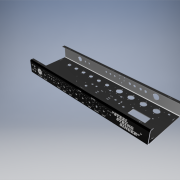
# Autodesk Inventor part: Main Enclosurewith silkscreen
Saved by Autodesk Inventor 2018.1 (Build 221171000, 171)
## iProperties
Created: 2017-10-21
Part Number: Main Enclosurewith silkscreen
Material: Aluminum 6061
Document SubType Name: Sheet Metal
Designer: RCCol
Density: 2.7 g/cm^3
Sheet Metal Rule: .125 thick aluminum
Appearance: Aluminum - Flat
Sheet Metal Width: 14.631 in
Sheet Metal Length: 26.500 in
Sheet Metal Area: 387.721 in^2
Flat Pattern Width: 37.1627 cm
Flat Pattern Length: 67.31 cm
Flat Pattern Area: 2501.42 cm^2
Author: RCCol
Autodesk Inventor part; units mm, degrees
ref_plane "YZ Plane" through (0, 0, 0) normal (1, 0, 0) x (0, 1, 0)
ref_plane "XZ Plane" through (0, 0, 0) normal (0, 1, 0) x (-1, 0, 0)
ref_plane "XY Plane" through (0, 0, 0) normal (0, 0, 1) x (1, 0, 0)
sketch "Sketch2" plane through (0, 0, 0) normal (0, 1, 0) x (-1, 0, 0)
  circle A0 centre (244.7036, -254.3608) radius 1.651
  circle A1 centre (234.6008, -260.133) radius 1.651
  circle A2 centre (193.9036, -270.2358) radius 9.525
  circle A3 centre (140.559, -225.1508) radius 1.65
  line L0 (-268.3747, -289.9675) -> (-268.3747, -293.6791)
  arc A4 (-268.3747, -289.9675) -> (-268.97, -289.3722) centre (-268.97, -289.9675) ccw
  line L1 (-271.0814, -289.3722) -> (-268.97, -289.3722)
  arc A5 (-271.0814, -289.3722) -> (-271.6767, -289.9675) centre (-271.0814, -289.9675) ccw
  line L2 (-271.6767, -293.6791) -> (-271.6767, -289.9675)
  arc A6 (-271.6767, -293.6791) -> (-271.0814, -294.2744) centre (-271.0814, -293.6791) ccw
  line L3 (-268.97, -294.2744) -> (-271.0814, -294.2744)
  arc A7 (-268.97, -294.2744) -> (-268.3747, -293.6791) centre (-268.97, -293.6791) ccw
  circle A8 centre (-298.0757, -244.2954) radius 1.651
  circle A9 centre (143.1036, -270.2358) radius 9.525
  line L4 (-268.3747, -249.9675) -> (-268.3747, -253.6791)
  arc A10 (-268.3747, -249.9675) -> (-268.97, -249.3722) centre (-268.97, -249.9675) ccw
  line L5 (-271.0814, -249.3722) -> (-268.97, -249.3722)
  arc A11 (-271.0814, -249.3722) -> (-271.6767, -249.9675) centre (-271.0814, -249.9675) ccw
  line L6 (-271.6767, -253.6791) -> (-271.6767, -249.9675)
  arc A12 (-271.6767, -253.6791) -> (-271.0814, -254.2744) centre (-271.0814, -253.6791) ccw
  line L7 (-268.97, -254.2744) -> (-271.0814, -254.2744)
  arc A13 (-268.97, -254.2744) -> (-268.3747, -253.6791) centre (-268.97, -253.6791) ccw
  circle A14 centre (143.1036, -254.3608) radius 1.651
  circle A15 centre (-285.3757, -224.1983) radius 3.175
  circle A16 centre (133.0008, -260.133) radius 1.651
  circle A17 centre (92.3036, -286.1108) radius 1.651
  circle A18 centre (202.3125, -144.8233) radius 1.651
  circle A19 centre (71.2868, -214.9908) radius 2.3813
  circle A20 centre (-285.3757, -147.9983) radius 3.175
  circle A21 centre (190.3125, -135.2983) radius 1.651
  circle A22 centre (92.3036, -254.3608) radius 1.651
  circle A23 centre (-174.7757, -281.3483) radius 1.651
  circle A24 centre (176.9125, -135.2983) radius 1.651
  circle A25 centre (42.134, -229.1208) radius 4.826
  arc A26 (-141.3747, -289.9675) -> (-141.97, -289.3722) centre (-141.97, -289.9675) ccw
  line L8 (-144.0814, -289.3722) -> (-141.97, -289.3722)
  arc A27 (-144.0814, -289.3722) -> (-144.6767, -289.9675) centre (-144.0814, -289.9675) ccw
  line L9 (-144.6767, -293.6791) -> (-144.6767, -289.9675)
  arc A28 (-144.6767, -293.6791) -> (-144.0814, -294.2744) centre (-144.0814, -293.6791) ccw
  line L10 (-141.97, -294.2744) -> (-144.0814, -294.2744)
  arc A29 (-141.97, -294.2744) -> (-141.3747, -293.6791) centre (-141.97, -293.6791) ccw
  line L11 (-141.3747, -289.9675) -> (-141.3747, -293.6791)
  circle A30 centre (157.8625, -135.2983) radius 1.651
  circle A31 centre (41.5036, -270.2358) radius 9.525
  circle A32 centre (16.734, -229.1208) radius 4.826
  circle A33 centre (-111.2757, -280.4425) radius 1.651
  circle A34 centre (-47.7757, -280.4425) radius 1.651
  circle A35 centre (-190.1257, -224.1983) radius 3.175
  arc A36 (-141.3747, -249.9675) -> (-141.97, -249.3722) centre (-141.97, -249.9675) ccw
  line L12 (-144.0814, -249.3722) -> (-141.97, -249.3722)
  arc A37 (-144.0814, -249.3722) -> (-144.6767, -249.9675) centre (-144.0814, -249.9675) ccw
  line L13 (-144.6767, -253.6791) -> (-144.6767, -249.9675)
  arc A38 (-144.6767, -253.6791) -> (-144.0814, -254.2744) centre (-144.0814, -253.6791) ccw
  line L14 (-141.97, -254.2744) -> (-144.0814, -254.2744)
  arc A39 (-141.97, -254.2744) -> (-141.3747, -253.6791) centre (-141.97, -253.6791) ccw
  line L15 (-141.3747, -249.9675) -> (-141.3747, -253.6791)
  circle A40 centre (-19.3992, -260.133) radius 1.651
  circle A41 centre (-79.5257, -271.8233) radius 15.1
  line L16 (-28.621, -217.7185) -> (-21.621, -217.7185)
  arc A42 (-28.621, -217.7185) -> (-28.621, -222.7185) centre (-28.621, -220.2185) ccw
  line L17 (-21.621, -222.7185) -> (-28.621, -222.7185)
  arc A43 (-21.621, -222.7185) -> (-21.621, -217.7185) centre (-21.621, -220.2185) ccw
  arc A44 (-77.8747, -249.9675) -> (-78.47, -249.3722) centre (-78.47, -249.9675) ccw
  line L18 (-80.5814, -249.3722) -> (-78.47, -249.3722)
  arc A45 (-80.5814, -249.3722) -> (-81.1767, -249.9675) centre (-80.5814, -249.9675) ccw
  line L19 (-81.1767, -253.6791) -> (-81.1767, -249.9675)
  arc A46 (-81.1767, -253.6791) -> (-80.5814, -254.2744) centre (-80.5814, -253.6791) ccw
  line L20 (-78.47, -254.2744) -> (-80.5814, -254.2744)
  arc A47 (-78.47, -254.2744) -> (-77.8747, -253.6791) centre (-78.47, -253.6791) ccw
  line L21 (-77.8747, -249.9675) -> (-77.8747, -253.6791)
  circle A48 centre (-99.2757, -246.7925) radius 1.65
  circle A49 centre (-35.7757, -248.38) radius 1.65
  circle A50 centre (-60.681, -232.1358) radius 1.65
  circle A51 centre (-47.7757, -248.38) radius 4.826
  circle A52 centre (-172.441, -232.1358) radius 1.65
  circle A53 centre (-10.2592, -172.0483) radius 6.35
  circle A54 centre (-83.8585, -220.2185) radius 2.65
  line L22 (-83.768, -202.6483) -> (-76.768, -202.6483)
  arc A55 (-83.768, -202.6483) -> (-83.768, -207.6483) centre (-83.768, -205.1483) ccw
  line L23 (-76.768, -207.6483) -> (-83.768, -207.6483)
  arc A56 (-76.768, -207.6483) -> (-76.768, -202.6483) centre (-76.768, -205.1483) ccw
  line L24 (-18.6805, -126.4483) -> (-11.6805, -126.4483)
  arc A57 (-18.6805, -126.4483) -> (-18.6805, -131.4483) centre (-18.6805, -128.9483) ccw
  line L25 (-11.6805, -131.4483) -> (-18.6805, -131.4483)
  arc A58 (-11.6805, -131.4483) -> (-11.6805, -126.4483) centre (-11.6805, -128.9483) ccw
  line L26 (-28.621, -135.1685) -> (-21.621, -135.1685)
  arc A59 (-28.621, -135.1685) -> (-28.621, -140.1685) centre (-28.621, -137.6685) ccw
  line L27 (-21.621, -140.1685) -> (-28.621, -140.1685)
  arc A60 (-21.621, -140.1685) -> (-21.621, -135.1685) centre (-21.621, -137.6685) ccw
  circle A61 centre (-160.0585, -201.043) radius 4.8
  circle A62 centre (-60.681, -143.2358) radius 1.65
  circle A63 centre (-134.6585, -168.6358) radius 2.65
  circle A64 centre (-172.441, -143.2358) radius 1.65
  line L28 (-83.768, -126.4483) -> (-76.768, -126.4483)
  arc A65 (-83.768, -126.4483) -> (-83.768, -131.4483) centre (-83.768, -128.9483) ccw
  line L29 (-76.768, -131.4483) -> (-83.768, -131.4483)
  arc A66 (-76.768, -131.4483) -> (-76.768, -126.4483) centre (-76.768, -128.9483) ccw
  circle A67 centre (-134.6585, -128.9483) radius 2.65
  line L30 (-132.1585, -137.9577) -> (-132.1585, -142.9577)
  arc A68 (-132.1585, -137.9577) -> (-137.1585, -137.9577) centre (-134.6585, -137.9577) ccw
  line L31 (-137.1585, -142.9577) -> (-137.1585, -137.9577)
  arc A69 (-137.1585, -142.9577) -> (-132.1585, -142.9577) centre (-134.6585, -142.9577) ccw
  circle A70 centre (-83.8585, -137.6685) radius 2.65
  circle A71 centre (-75.921, -137.6685) radius 2.65
  circle A72 centre (-85.1892, -172.0483) radius 6.35
  line L32 (-132.1585, -202.9264) -> (-132.1585, -207.9264)
  arc A73 (-132.1585, -202.9264) -> (-137.1585, -202.9264) centre (-134.6585, -202.9264) ccw
  line L33 (-137.1585, -207.9264) -> (-137.1585, -202.9264)
  arc A74 (-137.1585, -207.9264) -> (-132.1585, -207.9264) centre (-134.6585, -207.9264) ccw
  line L34 (-83.768, -191.9483) -> (-76.768, -191.9483)
  arc A75 (-83.768, -191.9483) -> (-83.768, -196.9483) centre (-83.768, -194.4483) ccw
  line L35 (-76.768, -196.9483) -> (-83.768, -196.9483)
  arc A76 (-76.768, -196.9483) -> (-76.768, -191.9483) centre (-76.768, -194.4483) ccw
  circle A77 centre (-40.416, -168.0008) radius 1.65
  circle A78 centre (-107.616, -213.8685) radius 4.8
  line L36 (-132.1585, -216.9358) -> (-132.1585, -221.9358)
  arc A79 (-132.1585, -216.9358) -> (-137.1585, -216.9358) centre (-134.6585, -216.9358) ccw
  line L37 (-137.1585, -221.9358) -> (-137.1585, -216.9358)
  arc A80 (-137.1585, -221.9358) -> (-132.1585, -221.9358) centre (-134.6585, -221.9358) ccw
  circle A81 centre (-75.921, -220.2185) radius 2.65
  circle A82 centre (-190.1257, -147.9983) radius 3.175
  line L38 (-18.6805, -191.9483) -> (-11.6805, -191.9483)
  arc A83 (-18.6805, -191.9483) -> (-18.6805, -196.9483) centre (-18.6805, -194.4483) ccw
  line L39 (-11.6805, -196.9483) -> (-18.6805, -196.9483)
  arc A84 (-11.6805, -196.9483) -> (-11.6805, -191.9483) centre (-11.6805, -194.4483) ccw
  line L40 (-196.4757, -155.6433) -> (-196.4757, -216.5533)
  arc A85 (-196.4757, -155.6433) -> (-199.6757, -152.4433) centre (-199.6757, -155.6433) ccw
  line L41 (-275.8257, -152.4433) -> (-199.6757, -152.4433)
  arc A86 (-275.8257, -152.4433) -> (-279.0257, -155.6433) centre (-275.8257, -155.6433) ccw
  line L42 (-279.0257, -216.5533) -> (-279.0257, -155.6433)
  arc A87 (-279.0257, -216.5533) -> (-275.8257, -219.7533) centre (-275.8257, -216.5533) ccw
  line L43 (-199.6757, -219.7533) -> (-275.8257, -219.7533)
  arc A88 (-199.6757, -219.7533) -> (-196.4757, -216.5533) centre (-199.6757, -216.5533) ccw
  circle A89 centre (-59.7757, -248.38) radius 1.65
  line L44 (-18.6805, -202.6483) -> (-11.6805, -202.6483)
  arc A90 (-18.6805, -202.6483) -> (-18.6805, -207.6483) centre (-18.6805, -205.1483) ccw
  line L45 (-11.6805, -207.6483) -> (-18.6805, -207.6483)
  arc A91 (-11.6805, -207.6483) -> (-11.6805, -202.6483) centre (-11.6805, -205.1483) ccw
  circle A92 centre (-111.2757, -246.7925) radius 4.826
  circle A93 centre (-40.416, -225.1508) radius 1.65
  circle A94 centre (-123.2757, -246.7925) radius 1.65
  circle A95 centre (-9.2964, -254.3608) radius 1.651
  circle A96 centre (-9.2964, -270.2358) radius 9.525
  circle A97 centre (-143.0257, -271.8233) radius 15.1
  circle A98 centre (144.4625, -135.2983) radius 1.651
  circle A99 centre (31.4008, -260.133) radius 1.651
  circle A100 centre (-179.9657, -245.0256) radius 1.651
  circle A101 centre (0.8064, -280.3386) radius 1.651
  arc A102 (-77.8747, -289.9675) -> (-78.47, -289.3722) centre (-78.47, -289.9675) ccw
  line L46 (-80.5814, -289.3722) -> (-78.47, -289.3722)
  arc A103 (-80.5814, -289.3722) -> (-81.1767, -289.9675) centre (-80.5814, -289.9675) ccw
  line L47 (-81.1767, -293.6791) -> (-81.1767, -289.9675)
  arc A104 (-81.1767, -293.6791) -> (-80.5814, -294.2744) centre (-80.5814, -293.6791) ccw
  line L48 (-78.47, -294.2744) -> (-80.5814, -294.2744)
  arc A105 (-78.47, -294.2744) -> (-77.8747, -293.6791) centre (-78.47, -293.6791) ccw
  line L49 (-77.8747, -289.9675) -> (-77.8747, -293.6791)
  circle A106 centre (53.7855, -199.9147) radius 6.35
  line L50 (-204.8747, -249.9675) -> (-204.8747, -253.6791)
  arc A107 (-204.8747, -249.9675) -> (-205.47, -249.3722) centre (-205.47, -249.9675) ccw
  line L51 (-207.5814, -249.3722) -> (-205.47, -249.3722)
  arc A108 (-207.5814, -249.3722) -> (-208.1767, -249.9675) centre (-207.5814, -249.9675) ccw
  line L52 (-208.1767, -253.6791) -> (-208.1767, -249.9675)
  arc A109 (-208.1767, -253.6791) -> (-207.5814, -254.2744) centre (-207.5814, -253.6791) ccw
  line L53 (-205.47, -254.2744) -> (-207.5814, -254.2744)
  arc A110 (-205.47, -254.2744) -> (-204.8747, -253.6791) centre (-205.47, -253.6791) ccw
  circle A111 centre (-206.5257, -271.8233) radius 15.1
  circle A112 centre (51.6064, -280.3386) radius 1.651
  circle A113 centre (82.2008, -260.133) radius 1.651
  circle A114 centre (92.3036, -270.2358) radius 9.525
  circle A115 centre (-285.3757, -129.8538) radius 1.5
  circle A116 centre (-238.2757, -244.2954) radius 1.651
  line L54 (-204.8747, -289.9675) -> (-204.8747, -293.6791)
  arc A117 (-204.8747, -289.9675) -> (-205.47, -289.3722) centre (-205.47, -289.9675) ccw
  line L55 (-207.5814, -289.3722) -> (-205.47, -289.3722)
  arc A118 (-207.5814, -289.3722) -> (-208.1767, -289.9675) centre (-207.5814, -289.9675) ccw
  line L56 (-208.1767, -293.6791) -> (-208.1767, -289.9675)
  arc A119 (-208.1767, -293.6791) -> (-207.5814, -294.2744) centre (-207.5814, -293.6791) ccw
  line L57 (-205.47, -294.2744) -> (-207.5814, -294.2744)
  arc A120 (-205.47, -294.2744) -> (-204.8747, -293.6791) centre (-205.47, -293.6791) ccw
  circle A121 centre (98.653, -179.9637) radius 2.3813
  circle A122 centre (102.4064, -280.3386) radius 1.651
  circle A123 centre (-238.2757, -280.4425) radius 1.651
  circle A124 centre (110.892, -194.8109) radius 2.3813
  circle A125 centre (-270.0257, -271.8233) radius 15.1
  circle A126 centre (221.3625, -144.8233) radius 1.651
  circle A127 centre (140.559, -168.0008) radius 1.65
  circle A128 centre (153.2064, -280.3386) radius 1.651
  circle A129 centre (183.8008, -260.133) radius 1.651
  circle A130 centre (-294.9007, -286.7925) radius 1.651
  circle A131 centre (204.0064, -280.3386) radius 1.651
  circle A132 centre (244.7036, -270.2358) radius 9.525
  circle A133 centre (254.8064, -280.3386) radius 1.651
  line L58 (322.2625, -312.7375) -> (-350.8375, -312.7375)
  line L59 (-350.8375, -312.7375) -> (-350.8375, -96.8375)
  line L60 (-350.8375, -96.8375) -> (322.2625, -96.8375)
  line L61 (322.2625, -96.8375) -> (322.2625, -312.7375)
  circle A134 centre (317.5, -133.35) radius 2.667
  circle A135 centre (317.5, -140.6906) radius 1.5875
  circle A136 centre (317.5, -126.0094) radius 1.5875
  circle A137 centre (317.5, -273.05) radius 2.667
  circle A138 centre (317.5, -280.3906) radius 1.5875
  circle A139 centre (317.5, -265.7094) radius 1.5875
  point P0 (0, 0)
  dimension "d2" = 673.1
  dimension "d3" = 215.9
  measures "d2" distance of L59.end L60.end
  measures "d3" distance of L58.end L59.end
extrude "Plate1" add sketch "Sketch2" along normal blind 3.175 contours L58 L59 L60 L61 | A134 | A135 | A136 | A137 | A138 | A139
sketch "Sketch3" plane through (350.8375, 0, -100.0125) normal (0, 0, 1) x (1, 0, 0)
  line L0 (-673.1, 0) -> (0, 0)
  line L1 (0, 0) -> (0, 69.85)
  line L2 (0, 69.85) -> (-673.1, 69.85)
  line L3 (-673.1, 69.85) -> (-673.1, 0)
  constraints: 6 end point, 1 horizontal, 1 perpendicular, 1 vertical
edge flange "Flange1" height 69.85 angle 90 thickness 3.175 bend radius 3.175 thickness toward (0, 0, 1) relief tear relief width 3.175 relief depth 1.5875 edges at (14.2875, 3.175, -96.8375) wall of the first edge with corners at (-322.2625, 0, -100.0125) (350.8375, 0, -100.0125) (350.8375, 69.85, -100.0125) (-322.2625, 69.85, -100.0125)
bend "Bend1"
corner "Corner1"
sketch "Sketch4" plane through (-322.2625, 0, -309.5625) normal (0, 0, -1) x (-1, 0, 0)
  line L0 (-673.1, 0) -> (0, 0)
  line L1 (0, 0) -> (0, 69.85)
  line L2 (0, 69.85) -> (-673.1, 69.85)
  line L3 (-673.1, 69.85) -> (-673.1, 0)
  constraints: 6 end point, 1 horizontal, 1 perpendicular, 1 vertical
edge flange "Flange2" height 69.85 angle 90 thickness 3.175 bend radius 3.175 thickness toward (0, 0, -1) relief tear relief width 3.175 relief depth 1.5875 edges at (14.2875, 3.175, -312.7375) wall of the first edge with corners at (350.8375, 0, -309.5625) (-322.2625, 0, -309.5625) (-322.2625, 69.85, -309.5625) (350.8375, 69.85, -309.5625)
bend "Bend2"
corner "Corner2"
sketch "A$C2850429B" plane through (0, 0, 0) normal (0, 0, 1) x (1, 0, 0)
  circle A0 centre (0, 0) radius 1.778
sketch "A$C2850429B_1" plane through (0, 0, 0) normal (0, 0, 1) x (1, 0, 0)
  circle A0 centre (0, 0) radius 1.778
sketch "A$C2850429B_2" plane through (0, 0, 0) normal (0, 0, 1) x (1, 0, 0)
  circle A0 centre (0, 0) radius 1.778
sketch "Sketch9" plane through (-322.2625, 69.85, -96.8375) normal (0, 0, 1) x (1, 0, 0)
  circle A0 centre (31.75, -22.225) radius 4.7625
  circle A1 centre (69.85, -34.925) radius 4.7625
  circle A2 centre (139.7, -34.925) radius 3.175
  circle A3 centre (171.704, -34.925) radius 3.175
  circle A4 centre (241.3, -34.925) radius 4.7625
  circle A5 centre (641.35, -34.925) radius 3.9624
  circle A6 centre (355.6, -34.925) radius 4.7625
  circle A7 centre (501.65, -34.925) radius 3.175
  circle A8 centre (469.9, -34.925) radius 4.7625
  circle A9 centre (431.8, -34.925) radius 4.7625
  circle A10 centre (393.7, -34.925) radius 4.7625
  circle A11 centre (317.5, -34.925) radius 4.7625
  circle A12 centre (279.4, -34.925) radius 4.7625
  circle A13 centre (203.2, -34.925) radius 4.7625
  circle A14 centre (155.702, -34.925) radius 3.175
  circle A15 centre (107.95, -34.925) radius 4.7625
  circle A16 centre (31.75, -47.625) radius 4.7625
  circle A17 centre (31.75, -47.625) radius 4.7625
  circle A18 centre (107.95, -34.925) radius 4.7625
  circle A19 centre (155.702, -34.925) radius 3.175
  circle A20 centre (203.2, -34.925) radius 4.7625
  circle A21 centre (279.4, -34.925) radius 4.7625
  circle A22 centre (317.5, -34.925) radius 4.7625
  circle A23 centre (393.7, -34.925) radius 4.7625
  circle A24 centre (431.8, -34.925) radius 4.7625
  circle A25 centre (469.9, -34.925) radius 4.7625
  circle A26 centre (501.65, -34.925) radius 3.175
  circle A27 centre (355.6, -34.925) radius 4.7625
  circle A28 centre (641.35, -34.925) radius 3.9624
  circle A29 centre (241.3, -34.925) radius 4.7625
  circle A30 centre (171.704, -34.925) radius 3.175
  circle A31 centre (139.7, -34.925) radius 3.175
  circle A32 centre (69.85, -34.925) radius 4.7625
  circle A33 centre (31.75, -22.225) radius 4.7625
  line L0 (0, -63.5) -> (0, 0) projected
  line L1 (0, -6.35) -> (673.1013, -6.35) construction
  line L2 (673.1013, -6.35) -> (673.1013, -63.5001) construction
  line L3 (673.1013, -63.5001) -> (0, -63.5001) construction
  line L4 (0, -63.5001) -> (0, -6.35) construction
  point P0 (322.2625, -69.85)
  constraints: 34 centre point, 17 concentric, 14 equal radius, 1 point on line, 2 other
extrude "Cut1" cut sketch "Sketch9" against normal blind 3.175
sketch "Sketch10" plane through (-322.2625, 69.85, -312.7375) normal (0, 1, 0) x (1, 0, 0)
  point P0 (322.2625, -312.7375)
sketch "Sketch13" plane through (-322.2625, 66.675, -312.7375) normal (0, 1, 0) x (-1, 0, 0)
  line L0 (-673.1, 0) -> (0, 0)
  line L1 (0, 0) -> (0, 19.05)
  line L2 (0, 19.05) -> (-673.1, 19.05)
  line L3 (-673.1, 19.05) -> (-673.1, 0)
  constraints: 6 end point, 1 horizontal, 1 perpendicular, 1 vertical
edge flange "Flange9" height 19.05 angle 90 thickness 3.175 bend radius 3.175 thickness toward (0, 1, 0) relief tear relief width 3.175 relief depth 1.5875 edges at (14.2875, 69.85, -309.5625) wall of the first edge with corners at (350.8375, 66.675, -312.7375) (-322.2625, 66.675, -312.7375) (-322.2625, 66.675, -293.6875) (350.8375, 66.675, -293.6875)
bend "Bend9"
corner "Corner9"
sketch "Sketch14" plane through (350.8375, 66.675, -96.8375) normal (0, 1, 0) x (-1, 0, 0)
  line L0 (673.1, 0) -> (0, 0)
  line L1 (0, 0) -> (0, -19.05)
  line L2 (0, -19.05) -> (673.1, -19.05)
  line L3 (673.1, -19.05) -> (673.1, 0)
  constraints: 6 end point, 1 horizontal, 1 perpendicular, 1 vertical
edge flange "Flange10" height 19.05 angle 90 thickness 3.175 bend radius 3.175 thickness toward (0, 1, 0) relief tear relief width 3.175 relief depth 1.5875 edges at (14.2875, 69.85, -100.0125) wall of the first edge with corners at (-322.2625, 66.675, -96.8375) (350.8375, 66.675, -96.8375) (350.8375, 66.675, -115.8875) (-322.2625, 66.675, -115.8875)
bend "Bend10"
corner "Corner10"
sketch "Sketch16" plane through (350.4375, 76.9937, -312.7375) normal (0, 0, -1) x (-1, 0, 0)
  line L0 (222.9999, -47.2355) -> (221.4962, -47.2355)
  arc A0 (222.9999, -48.2515) -> (221.4962, -48.2515) centre (222.248, -42.0741) ccw
  line L1 (221.4962, -47.2355) -> (221.4962, -48.2515)
  line L2 (222.9999, -48.2515) -> (222.9999, -47.2355)
  circle A1 centre (279.3859, -41.5187) radius 3.2385
  circle A2 centre (304.7859, -25.6437) radius 3.2385
  circle A3 centre (279.3859, -25.6437) radius 3.2385
  circle A4 centre (304.7859, -41.5187) radius 3.2385
  circle A5 centre (292.0309, -57.3937) radius 3.2385
  line L3 (196.213, -45.3834) -> (196.213, -38.7648)
  line L4 (184.783, -45.3834) -> (184.783, -38.7648)
  arc A6 (184.783, -45.3834) -> (196.213, -45.3834) centre (190.498, -42.0741) ccw
  arc A7 (196.213, -38.7648) -> (184.783, -38.7648) centre (190.498, -42.0741) ccw
  circle A8 centre (114.298, -42.0741) radius 14.7574
  circle A9 centre (135.253, -42.0741) radius 1.778
  circle A10 centre (93.343, -42.0741) radius 1.778
  line L5 (170.813, -45.3834) -> (170.813, -38.7648)
  line L6 (159.383, -45.3834) -> (159.383, -38.7648)
  arc A11 (159.383, -45.3834) -> (170.813, -45.3834) centre (165.098, -42.0741) ccw
  arc A12 (170.813, -38.7648) -> (159.383, -38.7648) centre (165.098, -42.0741) ccw
  line L7 (248.3999, -47.2355) -> (246.8962, -47.2355)
  arc A13 (248.3999, -48.2515) -> (246.8962, -48.2515) centre (247.648, -42.0741) ccw
  line L8 (246.8962, -47.2355) -> (246.8962, -48.2515)
  line L9 (248.3999, -48.2515) -> (248.3999, -47.2355)
  circle A14 centre (333.375, -41.5187) radius 4.7625
  circle A15 centre (358.775, -41.5187) radius 4.7625
  circle A16 centre (384.175, -41.5187) radius 4.7625
  circle A17 centre (495.2698, -42.1586) radius 4.7625
  circle A18 centre (520.6698, -42.1586) radius 4.7625
  circle A19 centre (558.7698, -42.1586) radius 12.1031
  circle A20 centre (545.9682, -34.7164) radius 1.778
  circle A21 centre (571.5714, -34.7164) radius 1.778
  circle A22 centre (558.7698, -56.9668) radius 1.778
  line L10 (-0.4, -13.4937) -> (672.6999, -13.4937) projected
  line L11 (-0.4, -13.4937) -> (672.7013, -13.4937) construction
  line L12 (672.7013, -13.4937) -> (672.7013, -70.6439) construction
  line L13 (672.7013, -70.6439) -> (-0.4, -70.6439) construction
  line L14 (-0.4, -70.6439) -> (-0.4, -13.4937) construction
  point P0 (322.2625, -69.85)
  constraints: 23 centre point, 20 end point, 14 equal radius, 12 point on circle, 2 concentric, 2 other
extrude "Cut2" cut sketch "Sketch16" against normal blind 3.175
sketch "Sketch17" plane through (-322.2625, 69.85, -293.6875) normal (0, 1, 0) x (1, 0, 0)
  circle A0 centre (50.8, -184.15) radius 2.667
  circle A1 centre (58.1406, -184.15) radius 1.5875
  circle A2 centre (43.4594, -184.15) radius 1.5875
  circle A3 centre (336.55, -184.15) radius 2.667
  circle A4 centre (343.8906, -184.15) radius 1.5875
  circle A5 centre (329.2094, -184.15) radius 1.5875
  circle A6 centre (622.3, -184.15) radius 2.667
  circle A7 centre (629.6406, -184.15) radius 1.5875
  circle A8 centre (614.9594, -184.15) radius 1.5875
  point P0 (322.2625, -293.6875)
  constraints: 9 centre point, 7 equal radius
extrude "Cut3" cut sketch "Sketch17" against normal blind 3.175
sketch "Sketch18" plane through (-322.2625, 69.85, -293.6875) normal (0, 1, 0) x (1, 0, 0)
  circle A0 centre (50.8, 6.35) radius 2.667
  circle A1 centre (58.1406, 6.35) radius 1.5875
  circle A2 centre (43.4594, 6.35) radius 1.5875
  circle A3 centre (336.55, 6.35) radius 2.667
  circle A4 centre (343.8906, 6.35) radius 1.5875
  circle A5 centre (329.2094, 6.35) radius 1.5875
  circle A6 centre (622.3, 6.35) radius 2.667
  circle A7 centre (629.6406, 6.35) radius 1.5875
  circle A8 centre (614.9594, 6.35) radius 1.5875
  point P0 (322.2625, -293.6875)
  constraints: 9 centre point, 7 equal radius
extrude "Cut4" cut sketch "Sketch18" against normal blind 3.175
sketch "Sketch21" plane through (0, 3.175, 0) normal (0, 1, 0) x (1, 0, 0)
  point P0 (0, 0)
sketch "Sketch22" plane through (0, 3.175, 0) normal (0, 1, 0) x (1, 0, 0)
  circle A0 centre (342.9, 274.6375) radius 2.667
  circle A1 centre (342.9, 267.2969) radius 1.5875
  circle A2 centre (342.9, 281.9781) radius 1.5875
  circle A3 centre (342.9, 134.9375) radius 2.667
  circle A4 centre (342.9, 127.5969) radius 1.5875
  circle A5 centre (342.9, 142.2781) radius 1.5875
  circle A6 centre (-314.325, 274.6375) radius 2.667
  circle A7 centre (-314.325, 267.2969) radius 1.5875
  circle A8 centre (-314.325, 281.9781) radius 1.5875
  circle A9 centre (-314.325, 134.9375) radius 2.667
  circle A10 centre (-314.325, 127.5969) radius 1.5875
  circle A11 centre (-314.325, 142.2781) radius 1.5875
  circle A12 centre (315.9125, 288.925) radius 4.7625
  point P0 (0, 0)
  dimension "BendReliefDepth" = 1.5875
  constraints: 13 centre point
extrude "Cut6" cut sketch "Sketch22" against normal blind 3.175
decal "Decal1"
decal "Decal2"
equation "\"d65\" = Thickness"
equation "\"BendReliefDepth\" = 0.5 * Thickness"
equation "\"d4\" = Thickness"
equation "\"d5\" = BendReliefWidth"
equation "\"d6\" = BendReliefDepth"
equation "\"d7\" = MinimumRemnant"
equation "\"d8\" = TransitionRadius"
equation "\"d11\" = BendRadius"
equation "\"d12\" = CornerReliefSize"
equation "\"d13\" = GapSize"
equation "\"d14\" = JacobiRadiusSize"
equation "\"d15\" = BendReliefWidth"
equation "\"d16\" = BendReliefDepth"
equation "\"d17\" = MinimumRemnant"
equation "\"d18\" = TransitionRadius"
equation "\"d21\" = BendRadius"
equation "\"d22\" = CornerReliefSize"
equation "\"d23\" = GapSize"
equation "\"d24\" = JacobiRadiusSize"
equation "\"d87\" = BendReliefWidth"
equation "\"d88\" = BendReliefDepth"
equation "\"d89\" = MinimumRemnant"
equation "\"d90\" = TransitionRadius"
equation "\"d93\" = BendRadius"
equation "\"d94\" = CornerReliefSize"
equation "\"d95\" = GapSize"
equation "\"d96\" = JacobiRadiusSize"
equation "\"d97\" = BendReliefWidth"
equation "\"d98\" = BendReliefDepth"
equation "\"d99\" = MinimumRemnant"
equation "\"d100\" = TransitionRadius"
equation "\"d103\" = BendRadius"
equation "\"d104\" = CornerReliefSize"
equation "\"d105\" = GapSize"
equation "\"d106\" = JacobiRadiusSize"
equation "\"BendRadius\" = Thickness"
equation "\"BendReliefWidth\" = Thickness"
equation "\"CornerReliefSize\" = 4 * Thickness"
equation "\"TransitionRadius\" = BendRadius"
equation "\"JacobiRadiusSize\" = BendRadius"
equation "\"GapSize\" = Thickness"
equation "\"Thickness\" = 3.175"
equation "\"MinimumRemnant\" = 6.35"
body "Solid1"
